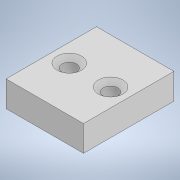
# Autodesk Inventor part: air delivery cover
Saved by Autodesk Inventor 2021.2 (Build 252289000, 289)
## iProperties
Created: 2021-07-12
Part Number: air delivery cover
Material: Generic
Document SubType Name: Modeling
Designer: jl4459
Density: 1 g/cm^3
Appearance: Default
Author: jl4459
Autodesk Inventor part; units mm, degrees
ref_plane "YZ Plane" through (0, 0, 0) normal (1, 0, 0) x (0, 1, 0)
ref_plane "XZ Plane" through (0, 0, 0) normal (0, 1, 0) x (-1, 0, 0)
ref_plane "XY Plane" through (0, 0, 0) normal (0, 0, 1) x (1, 0, 0)
sketch "Sketch1" plane through (0, 0, 0) normal (0, 1, 0) x (-1, 0, 0)
  line L0 (4.7625, 5.5626) -> (-4.7625, 5.5626)
  line L1 (-4.7625, 5.5626) -> (-4.7625, -5.5626)
  line L2 (-4.7625, -5.5626) -> (4.7625, -5.5626)
  line L3 (4.7625, -5.5626) -> (4.7625, 5.5626)
  point P0 (0, 0)
  dimension "d0" = 9.525
  dimension "d1" = 11.1252
  constraints: 8 end point, 2 parallel, 1 horizontal, 1 perpendicular
  measures "d0" distance of L2.end L1.end
  measures "d1" distance of L1.end L0.end
extrude "Extrusion1" add sketch "Sketch1" along normal blind 3.175
sketch "Sketch2" plane through (0, 3.175, 0) normal (0, 1, 0) x (1, 0, 0)
  line L0 (4.7625, 5.5626) -> (-4.7625, 5.5626) projected
  point P0 (0, 0)
  point P1 (-2.5457, 0)
  point P2 (2.5373, 0)
  dimension "d6" = 5.5626
  dimension "d14" = 5.5626
  measures "d6" distance from line of L0 point (2.537, 0)
  measures "d14" distance from line of L0 point (-2.546, 0)
hole "Hole1" at (2.5373, 3.175, 0) at (-2.5457, 3.175, 0) direction (0, -1, 0) diameter 1.778 end through all countersink diameter 3.0226 countersink angle 100 clearance for "Flat Head Machine Screw (82)" size "#0" standard "Ansi Unified Screw Threads"
body "Solid1"
